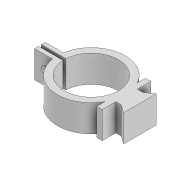
# Autodesk Inventor part: Acople Venturi
Saved by Autodesk Inventor 2022 (Build 260153000, 153)
## iProperties
Created: 2022-10-25
Part Number: Acople Venturi
Material: Generic
Document SubType Name: Modeling
Designer: ADMIN
Density: 1 g/cm^3
Appearance: Default
Author: ADMIN
## iProperties of the stored document Acople marcador_3DPrint.ipt
Created: 2022-10-25
Part Number: Acople marcador_3DPrint
Material: Generic
Document SubType Name: Modeling
Designer: ADMIN
Density: 1 g/cm^3
Appearance: Default
Author: ADMIN
Autodesk Inventor part; units mm, degrees
ref_plane "YZ Plane" through (0, 0, 0) normal (1, 0, 0) x (0, 1, 0)
ref_plane "XZ Plane" through (0, 0, 0) normal (0, 1, 0) x (-1, 0, 0)
sketch "Sketch1" plane through (0, 0, 0) normal (0, 1, 0) x (-1, 0, 0)
  line L0 (-0.116, 7.8509) -> (-0.116, -0.1491)
  line L1 (-0.116, -0.1491) -> (-3.116, -2.1491)
  line L2 (-3.116, -2.1491) -> (-3.116, 9.8509)
  line L3 (-0.116, 7.8509) -> (-3.116, 9.8509)
  line L4 (-0.116, 7.8509) -> (1.884, 7.8509)
  line L5 (1.884, 7.8509) -> (1.884, -0.1491)
  line L6 (1.884, -0.1491) -> (-0.116, -0.1491)
  point P0 (0, 0)
  dimension "d0" = 8
  dimension "d1" = 12
  dimension "d3" = 3
  dimension "d5" = 2
  dimension "d8" = 2
  constraints: 14 end point, 1 horizontal, 1 parallel, 1 perpendicular, 1 vertical
  measures "d0" distance of L0.start L0.end
  measures "d1" distance of L1.end L2.end
  measures "d3" distance between parallel lines of L2 L0
  measures "d5" vertical distance of L1.end L0.end
  measures "d8" distance of L0.start L4.end
extrude "Extrusion1" add sketch "Sketch1" along normal blind 10
ref_plane "Work Plane1" through (0, 5, 0) normal (0, 1, 0) x (1, 0, 0)
sketch "Sketch2" plane through (0, 5, 0) normal (0, 1, 0) x (1, 0, 0)
  circle A0 centre (-14.884, -3.8509) radius 12.5
  line L0 (-3.884, 5.1491) -> (-1.884, 5.1491)
  line L1 (-1.884, 5.1491) -> (-1.884, -12.8509)
  line L2 (-1.884, -12.8509) -> (-3.884, -12.8509)
  line L3 (-3.884, -12.8509) -> (-3.884, 5.1491)
  line L4 (3.116, -9.8509) -> (3.116, 2.1491) projected
  line L5 (0.116, -7.8509) -> (3.116, -9.8509) projected
  line L6 (-1.884, -7.8509) -> (0.116, -7.8509) projected
  line L7 (-1.884, 0.1491) -> (-1.884, -7.8509) projected
  line L8 (0.116, 0.1491) -> (-1.884, 0.1491) projected
  line L9 (3.116, 2.1491) -> (0.116, 0.1491) projected
  line L10 (3.116, -9.8509) -> (3.116, 2.1491) projected
  line L11 (0.116, -7.8509) -> (3.116, -9.8509) projected
  line L12 (-1.884, -7.8509) -> (0.116, -7.8509) projected
  line L13 (-1.884, 0.1491) -> (-1.884, -7.8509) projected
  line L14 (0.116, 0.1491) -> (-1.884, 0.1491) projected
  line L15 (3.116, 2.1491) -> (0.116, 0.1491) projected
  circle A1 centre (-14.884, -3.8509) radius 10
  line L16 (-29.8977, -3.3509) -> (-24.5183, -3.3509)
  line L17 (-24.5183, -3.3509) -> (-24.5183, -4.3509)
  line L18 (-24.5183, -4.3509) -> (-33.884, -4.3509)
  line L19 (-33.884, -4.3509) -> (-33.884, -1.5714)
  line L20 (-29.8977, -3.3509) -> (-33.884, -3.3509)
  line L21 (-33.884, -4.3509) -> (-33.884, -5.8509)
  line L22 (-33.884, -5.8509) -> (-24.682, -5.8509)
  line L23 (-33.884, -3.3509) -> (-33.884, -1.8509)
  line L24 (-33.884, -1.8509) -> (-24.682, -1.8509)
  point P0 (0, 0)
  point P1 (-27.223, -1.8509)
  point P2 (-24.8715, -3.3509)
  point P3 (-24.8715, -4.3509)
  point P4 (-27.223, -5.8509)
  point P5 (-3.884, -9.7881)
  point P6 (-3.884, 2.0862)
  point P7 (-27.374, -4.3509)
  point P8 (-27.374, -3.3509)
  point P9 (-1.884, -7.3509)
  point P10 (-1.884, -0.3509)
  point P11 (-3.884, -3.8509)
  dimension "d9" = 25
  dimension "d10" = 0
  dimension "d11" = 5
  dimension "d12" = 5
  dimension "d13" = 2
  dimension "d14" = 9
  dimension "d15" = 20
  dimension "d16" = 13
  dimension "d17" = 1
  dimension "d18" = 1.5
  dimension "d19" = 1.5
  dimension "d26" = 0.5
  dimension "d27" = 19
  constraints: 26 end point, 7 perpendicular, 2 centre point, 2 horizontal, 2 parallel, 2 point on circle, 2 point on line, 1 coincident, 1 vertical
  measures "d9" diameter of A0
  measures "d10" distance between parallel lines of L7 L1
  measures "d11" distance of L6.start L1.end
  measures "d12" distance from line of L8 L0.end
  measures "d13" distance of L0.start L0.end
  measures "d14" distance from line of L0 A0.centre
  measures "d15" diameter of A1
  measures "d16" distance from line of L7 A0.centre
  measures "d17" distance of L16.end L17.end
  measures "d18" distance of L18.end L21.end
  measures "d19" distance of L20.end L23.end
  measures "d26" vertical distance of A0.centre L17.end
  measures "d27" distance from line of A1.centre L21
extrude "Extrusion2" add sketch "Sketch2" along normal mid plane 10 contours A0 L3 | A0 L3 L0 L1 L2 | L3 A0 L22 A1 L24 | L24 A1 L16 A0 | A0 L16 L20 L19 L24 | L22 L21 L18 A0 | A0 L18 A1 L22
sketch "Sketch3" plane through (-27.223, 10, 1.8509) normal (0, 0, -1) x (-1, 0, 0)
  circle A0 centre (2.661, -4.9576) radius 1.5
  line L0 (0, 0) -> (6.661, 0) projected
  line L1 (0, -10) -> (0, 0) projected
  line L2 (6.661, -10) -> (0, -10) projected
  line L3 (6.661, -10) -> (6.661, 0) projected
  point P0 (-27.223, -10)
  dimension "d22" = 3
  dimension "d28" = 4
  constraints: 1 centre point
  measures "d22" diameter of A0
  measures "d28" distance from line of A0.centre L3
extrude "Extrusion3" cut sketch "Sketch3" against normal blind 10 contours A0
equation "\"d12\" = d11"
body "Solid1"
